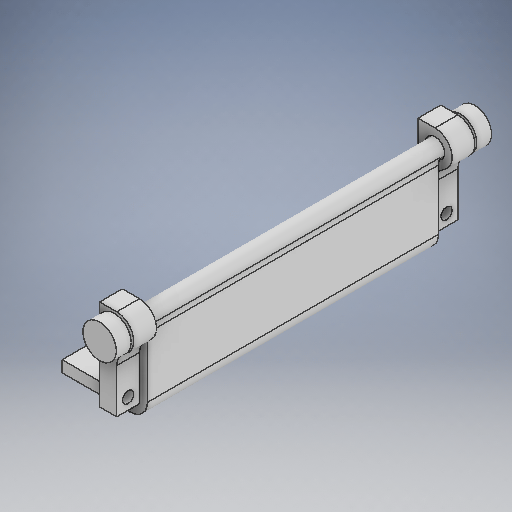
# Autodesk Inventor part: RP5_40pins_cover
Saved by Autodesk Inventor 2026.1 (Build 301233000, 233)
## iProperties
Created: 2025-12-16
Part Number: RP5_40pins_cover
Material: Generic
Document SubType Name: Modeling
Designer: emanuel
Density: 1 g/cm^3
Appearance: Default
Author: emanuel
Autodesk Inventor part; units mm, degrees
ref_plane "YZ Plane" through (0, 0, 0) normal (1, 0, 0) x (0, 1, 0)
ref_plane "XZ Plane" through (0, 0, 0) normal (0, 1, 0) x (-1, 0, 0)
ref_plane "XY Plane" through (0, 0, 0) normal (0, 0, 1) x (1, 0, 0)
sketch "Sketch1" plane through (0, 0, 0) normal (1, 0, 0) x (0, 1, 0)
  line L0 (0, 0) -> (0, -56)
  circle A0 centre (0, 0) radius 1
  circle A1 centre (0, -56) radius 1
  line L1 (0, 0) -> (-2, 0)
  line L2 (-2, 0) -> (-2, -2)
  line L3 (-2, -2) -> (0, -2)
  line L4 (0, -2) -> (0, 0)
  line L5 (0, -56) -> (-2, -56)
  line L6 (-2, -56) -> (-2, -54)
  line L7 (-2, -54) -> (0, -54)
  line L8 (0, -54) -> (0, -56)
  line L9 (-2, -54) -> (8, -54)
  line L10 (8, -54) -> (8, -2)
  line L11 (8, -2) -> (-2, -2)
  line L12 (-2, -2) -> (-2, -54)
  line L13 (0, 0) -> (-2, 0)
  line L14 (-2, 0) -> (-2, 2)
  line L15 (-2, 2) -> (0, 2)
  line L16 (0, 2) -> (0, 0)
  line L17 (-2, 2) -> (14, 2)
  line L18 (14, 2) -> (14, -58)
  line L19 (14, -58) -> (-2, -58)
  line L20 (-2, -58) -> (-2, 2)
  line L21 (8, -2) -> (14, -2)
  line L22 (14, -2) -> (14, -54)
  line L23 (14, -54) -> (8, -54)
  line L24 (8, -54) -> (8, -2)
  dimension "d0" = 56
  dimension "d1" = 2
  dimension "d2" = 2
  dimension "d3" = 2
  dimension "d4" = 2
  dimension "d5" = 2
  dimension "d6" = 2
  dimension "d7" = 10
  dimension "d8" = 2
  dimension "d9" = 2
  dimension "d10" = 16
  dimension "d11" = 60
  constraints: 50 end point, 12 parallel, 6 horizontal, 6 perpendicular, 2 centre point, 2 coincident, 2 point on line, 1 vertical
  measures "d0" distance of L0.start L0.end
  measures "d1" diameter of A0
  measures "d2" diameter of A1
  measures "d3" distance of L3.end L2.end
  measures "d4" distance of L2.end L1.end
  measures "d5" distance of L6.end L7.end
  measures "d6" distance of L5.end L6.end
  measures "d7" distance of L11.end L10.end
  measures "d8" distance of L14.end L15.end
  measures "d9" distance of L13.end L14.end
  measures "d10" distance of L18.end L19.end
  measures "d11" distance of L17.end L18.end
extrude "Extrusion1" add sketch "Sketch1" along normal blind 3 contours L3 L2 L1 A0 L0 | L0 A0 L16 L17 L18 L21 L11 | L9 L23 L18 L19 L20 L5 A1 L0 | L0 A1 L5 L6 L7 | L1 L14 L15 L16 A0
sketch "Sketch2" plane through (0, -2, 2) normal (0, 0, 1) x (1, 0, 0)
  line L0 (0, 0) -> (3, 0) projected
  line L1 (3, 0) -> (3, 10)
  line L2 (3, 16) -> (3, 0) projected
  line L3 (3, 10) -> (3, 13)
  circle A0 centre (3, 13) radius 1.7
  line L4 (0, 16) -> (3, 16) projected
  circle A1 centre (3, 13) radius 3
  point P0 (0, 2)
  point P1 (3, 10)
  point P2 (3, 14.7)
  point P3 (3, 11.3)
  dimension "d14" = 10
  dimension "d15" = 3
  dimension "d16" = 3.4
  constraints: 4 end point, 2 coincident, 2 point on line, 1 centre point, 3 other
  measures "d14" distance of L0.end L1.end
  measures "d15" distance of L1.end L3.end
  measures "d16" diameter of A0
extrude "Extrusion2" cut sketch "Sketch2" against normal blind 60 contours A1 L2 A0 | L2 A0 picked at (5.1258, 11.5893) picked at (2.8644, 11.8831)
extrude "Extrusion3" add sketch "Sketch2" against normal blind 60 contours A1 L2 A0 picked at (5.1258, 11.5893)
extrude "Extrusion4" cut sketch "Sketch1" along normal blind 60 contours L11 L10 L9 L0 | L21 L18 L23 L10
fillet "Fillet1" radius 3 2 edges at (3, 8, 0) (3, 8, -56)
sketch "Sketch3" plane through (0, -2, 2) normal (0, 0, 1) x (1, 0, 0)
  circle A0 centre (3, 13) radius 1.7 projected
  circle A1 centre (3, 13) radius 1.45
  point P0 (0, 2)
  dimension "d24" = 2.9
  constraints: 1 centre point, 1 coincident
  measures "d24" diameter of A1
extrude "Extrusion5" add sketch "Sketch3" along normal blind 3 and the other way blind 63 contours A1
sketch "Sketch4" plane through (3, 11, 5) normal (0, 0, 1) x (1, 0, 0)
  circle A0 centre (0, 0) radius 2.95
  point P0 (-3, -11)
  dimension "d29" = 5.9
  constraints: 1 centre point
  measures "d29" diameter of A0
extrude "Extrusion6" add sketch "Sketch4" against normal blind 2.6
sketch "Sketch5" plane through (3, 11, -61) normal (0, 0, -1) x (-1, 0, 0)
  circle A0 centre (0, 0) radius 1.45 projected
  circle A1 centre (0, 0) radius 2.95
  point P0 (3, -11)
  dimension "d32" = 5.9
  constraints: 1 centre point, 1 coincident
  measures "d32" diameter of A1
extrude "Extrusion7" add sketch "Sketch5" against normal blind 2.6
sketch "Sketch6" plane through (3, 0, 0) normal (1, 0, 0) x (0, 0, -1)
  line L0 (2, -2) -> (2, 5.8038) projected
  line L1 (2, -2) -> (2.4, -2)
  line L2 (2.4, -2) -> (53.6, -2)
  line L3 (2.4, -2) -> (53.6, -2)
  line L4 (53.6, -2) -> (53.6, 10.8701)
  line L5 (53.6, 10.8701) -> (2.4, 10.8701)
  line L6 (2.4, 10.8701) -> (2.4, -2)
  line L7 (2.4, -2) -> (53.6, -2)
  line L8 (53.6, -2) -> (53.6, -4.5)
  line L9 (53.6, -4.5) -> (2.4, -4.5)
  line L10 (2.4, -4.5) -> (2.4, -2)
  point P0 (0, 0)
  dimension "d35" = 0.4
  dimension "d36" = 51.2
  dimension "d37" = 2.5
  constraints: 20 end point, 4 parallel, 3 horizontal, 2 perpendicular, 2 point on line
  measures "d35" distance of L0.start L1.end
  measures "d36" distance of L1.end L2.end
  measures "d37" distance of L7.end L8.end
extrude "Extrusion8" add sketch "Sketch6" along normal mid plane 2
sketch "Sketch7" plane through (2, 0, 0) normal (-1, 0, 0) x (0, 0, 1)
  line L0 (-53.6, -4.5) -> (-2.4, -4.5) projected
  line L1 (-53.6, -4.5) -> (-2.4, -4.5)
  line L2 (-2.4, -4.5) -> (-2.4, -2.5)
  line L3 (-2.4, -2.5) -> (-53.6, -2.5)
  line L4 (-53.6, -2.5) -> (-53.6, -4.5)
  point P0 (0, 0)
  dimension "d40" = 2
  constraints: 8 end point, 2 parallel, 1 horizontal, 1 perpendicular
  measures "d40" distance of L2.end L1.end
extrude "Extrusion9" add sketch "Sketch7" along normal blind 13
fillet "Fillet2" radius 3 2 edges at (2, -2.5, -28) (4, -4.5, -28)
fillet "Fillet3" radius 3 2 edges at (4, 9.95, -28) (2, 9.95, -28)
body "Solid1"
